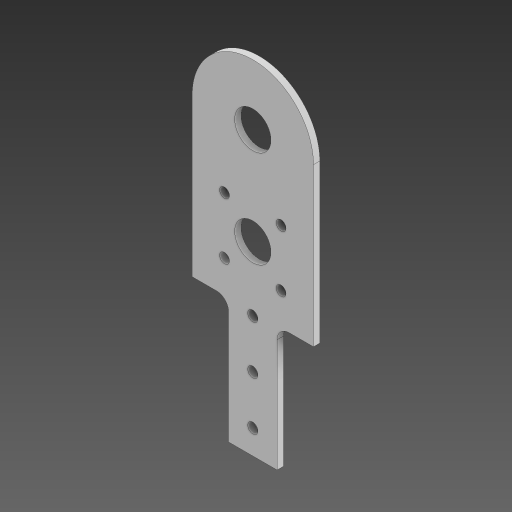
# Autodesk Inventor part: wrist plate 2
Saved by Autodesk Inventor 2024 (Build 280153000, 153)
## iProperties
Created: 2023-11-09
Part Number: wrist plate 2
Material: Generic
Document SubType Name: Modeling
Designer: ellen
Density: 1 g/cm^3
Appearance: Default
Author: ellen
Autodesk Inventor part; units mm, degrees
ref_plane "YZ Plane" through (0, 0, 0) normal (1, 0, 0) x (0, 1, 0)
ref_plane "XZ Plane" through (0, 0, 0) normal (0, 1, 0) x (-1, 0, 0)
ref_plane "XY Plane" through (0, 0, 0) normal (0, 0, 1) x (1, 0, 0)
sketch "Sketch1" plane through (0, 0, 0) normal (0, 0, 1) x (1, 0, 0)
  line L0 (63.5, 1.905) -> (63.5, 128.905)
  line L1 (63.5, 128.905) -> (0, 128.905)
  line L2 (0, 128.905) -> (0, 41.0985)
  circle A0 centre (31.75, 97.155) radius 9.5
  circle A1 centre (31.75, 46.355) radius 9.5
  circle A2 centre (31.75, 12.7) radius 2.6543
  line L3 (19.05, 0) -> (19.05, 14.605)
  line L4 (19.05, 25.4) -> (44.45, 25.4)
  line L5 (44.45, 25.4) -> (44.45, 0)
  line L6 (31.75, 0) -> (31.75, 128.905)
  circle A3 centre (31.75, -12.7) radius 2.6543
  circle A4 centre (31.75, -38.1) radius 2.6543
  line L7 (44.45, 0) -> (44.45, -50.8)
  line L8 (44.45, -50.8) -> (19.05, -50.8)
  line L9 (19.05, -50.8) -> (19.05, 0)
  line L10 (0, 41.0985) -> (0, 27.305)
  line L11 (63.5, 14.605) -> (0, 14.605)
  line L12 (0, 14.605) -> (0, 27.305)
  point P0 (0, 0)
  point P1 (63.5, 27.305)
  point P2 (44.45, 14.605)
  point P3 (31.75, -50.8)
  dimension "d0" = 63.5
  dimension "d1" = 127
  dimension "d3" = 116.205
  dimension "d4" = 31.75
  dimension "d5" = 82.55
  dimension "d12" = 19
  dimension "d13" = 19
  dimension "d14" = 5.3086
  dimension "d29" = 25.4
  dimension "d30" = 25.4
  dimension "d31" = 25.4
  dimension "d32" = 25.4
  dimension "d33" = 50.8
  dimension "d36" = 12.7
  constraints: 26 end point, 5 centre point, 3 perpendicular, 3 point on line, 3 vertical, 2 equal radius, 2 midpoint, 1 collinear, 1 horizontal, 1 parallel, 1 other
  measures "d0" distance of L1.end L0.end
  measures "d1" distance of L0.end L0.start
  measures "d3" distance from line of L1 A2.centre
  measures "d4" distance from line of L1 A0.centre
  measures "d5" distance from line of L1 A1.centre
  measures "d12" diameter of A0
  measures "d13" diameter of A1
  measures "d14" diameter of A2
  measures "d29" distance of L3.start L4.start
  measures "d30" distance of L4.start L4.end
  measures "d31" distance of A3.centre A2.centre
  measures "d32" distance of A4.centre A3.centre
  measures "d33" distance of L5.end L7.end
  measures "d36" distance of point (31.75, -50.8) A4.centre
extrude "Extrusion1" add sketch "Sketch1" along normal blind 3.302 contours L11 L5 L4 L6 A1 A0 L1 L0 | L11 A2 L6 L4 L5 | L5 L7 L8 L9 L3 L11 A2 | L6 A0 A1 A2 L11 L12 L10 L2 L1
fillet "Fillet1" radius 31.75 1 edges at (63.5, 128.905, 1.651)
fillet "Fillet2" radius 31.75 1 edges at (0, 128.905, 1.651)
sketch "Sketch3" plane through (0, 0, 3.302) normal (0, 0, 1) x (1, 0, 0)
  circle A0 centre (31.75, 46.355) radius 9.5 projected
  circle A1 centre (31.75, 46.355) radius 20.955
  line L0 (31.75, 46.355) -> (4.2793, 73.8257)
  line L1 (4.2793, 73.8257) -> (54.0042, 24.1008)
  line L2 (31.75, 46.355) -> (57.6977, 72.3027)
  line L3 (31.75, 46.355) -> (13.6103, 28.2153)
  line L4 (31.75, 46.355) -> (57.4034, 46.355) construction
  point P0 (0, 0)
  point P1 (46.5674, 61.1724)
  point P2 (46.5674, 31.5376)
  point P3 (16.9326, 61.1724)
  point P4 (16.9326, 31.5376)
  dimension "d16" = 41.91
  dimension "d28" = 135
  constraints: 10 end point, 6 point on line, 4 point on circle, 1 centre point, 1 coincident, 1 equal length, 1 horizontal
  measures "d16" diameter of A1
  measures "d28" angle of L3 L4
hole "Hole1" at (46.5674, 61.1724, 3.302) at (46.5674, 31.5376, 3.302) at (16.9326, 61.1724, 3.302) at (16.9326, 31.5376, 3.302) direction (0, 0, -1) diameter 5.1054 depth 16.256 tip angle 118 clearance for "Flat Head Machine Screw (82)" size "#10" standard "Ansi Unified Screw Threads"
fillet "Fillet5" radius 6.35 1 edges at (19.05, 14.605, 1.651)
fillet "Fillet6" radius 6.35 1 edges at (44.45, 14.605, 1.651)
equation "\"d13\" = d12"
body "Solid1"
